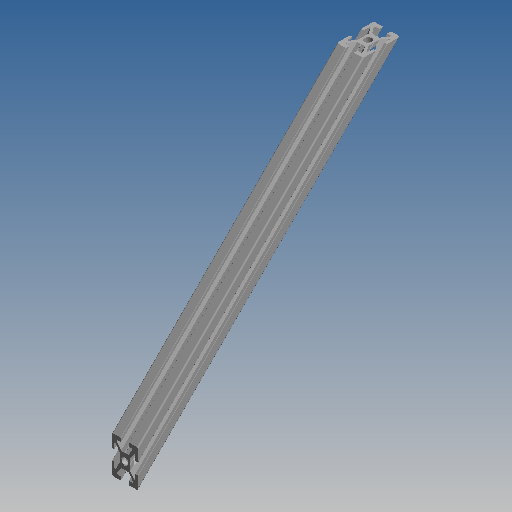
# Autodesk Inventor part: HFBL5-2020-200_
Saved by Autodesk Inventor 2020 (Build 240168000, 168)
## iProperties
Part Number: HFBL5-2020-200_
Material: 一般
Catalog Web Link: www.cadenas.de
Description: HFBL5_-Brackets HFS5 Frame Brackets for Reinforcement
Vendor: MISUMI
Document SubType Name: Modeling
Designer: partserver
Manufacturer: MISUMI
Mass: 47.3793 g
Surface Area: 458.252 cm^2
Volume: 47.3793 cm^3
Density: 1 g/cm^3
Appearance: PSOLRGB-192-192-192
Category: PARTsolutions
Company: MISUMI
PSOL_IDENT_0: {$CADENAS_DATA\23d-libs\misumi\metric\38_al_extrusions_blackets\5\hfbl5.prj},176 {VTYP=3D},{NB=HFBL5
PSOL_IDENT_1: -2020-200_},{LINA=HFBL5-2020-200_},{NN=HFBL5_},{DATE=24.04.2017 10:22:18},{GEOMDATE=30.01.2015 00:00
PSOL_IDENT_2: :00},{VERSION=},{LINEID=10},{WBVAR=L,ALT},{WBNUMERIC=L}  {NB=HFBL5-2020-200_},{LINA=HFBL5-2020-200_}
PSOL_IDENT_3: ,{KT=1},{PN=HFBL5-2020-200},{TP=HFBL5},{NO=2020},{TYPE=HFBL5},{MAT=A6N01SS-T5},{ST=Alumite Treatment
PSOL_IDENT_4: (No surface treatment on the side cut at 45 degree and  Counterbore type)},{FEAT=4 Slots},{L=200},{
PSOL_IDENT_5: LTOL=+/- 0.5},{MASS=0.50},{SA=153},{GMILX=0.57x10^4},{GMILY=0.57x10^4},{WIDTH=20},{HEIGHT=20},{TAPDE
PSOL_IDENT_6: PTH=15},{TAPSTART=0},{DRILLLENGTH=0},{DRILLDIA=4.2},{TAPPOSHOR=0},{TAPPOSVER=0},{VER=1},{DIM=1},{CLF=
PSOL_IDENT_7: HFS5-2020},{ALT3=},{AB=CBM5-8},{ABQ=2},{AN=HNTT5-5},{ANQ=2},{ALT=}
NB: HFBL5-2020-200_
NN: HFBL5_
NT: Brackets HFS5 Frame Brackets for Reinforcement
NBSYN: $PN._
LINA: HFBL5-2020-200_
CATALOG: Misumi
PN: HFBL5-2020-200
NO: 2020
MAT: A6N01SS-T5 Aluminum Alloy
ST: Alumite Treatment (No surface treatment on the side cut at 45 degree and  Counterbore type)
L: 200
WIDTH: 20
AB: CBM5-8
ABQ: 2
AN: HNTT5-5
ANQ: 2
ALT: w/o Set of Applicable Bolt and Nut
SUPPLIER: MISUMI
ARTICLENO: HFBL5-2020-200_
BOMINFO: HFBL5-2020-200_
CREATOR: CADENAS GmbH
Title: HFBL5-2020-200_
Author: Cadenas PARTsolutions
Comments: Brackets HFS5 Frame Brackets for Reinforcement
Autodesk Inventor part; units mm, degrees
sketch "Sketch_1" plane through (0, 0, 0) normal (0, -0.7071068, 0.7071068) x (1, 0, 0)
  arc A0 (-10, 134.7214) -> (-9.7, 134.4214) centre (-9.7, 134.7214) ccw
  line L0 (-9.7, 134.4214) -> (-8, 134.4214)
  line L1 (-8, 134.4214) -> (-8, 137.4214)
  line L2 (-8, 137.4214) -> (-7.0607, 137.4214)
  line L3 (-7.0607, 137.4214) -> (-4, 134.3607)
  line L4 (-4, 134.3607) -> (-4, 131.7214)
  line L5 (-4, 131.7214) -> (-3.7, 131.4214)
  line L6 (-3.7, 131.4214) -> (-4, 131.1214)
  line L7 (-4, 131.1214) -> (-4, 128.482)
  line L8 (-4, 128.482) -> (-7.0607, 125.4214)
  line L9 (-7.0607, 125.4214) -> (-8, 125.4214)
  line L10 (-8, 125.4214) -> (-8, 128.4214)
  line L11 (-8, 128.4214) -> (-9.7, 128.4214)
  arc A1 (-9.7, 128.4214) -> (-10, 128.1214) centre (-9.7, 128.1214) ccw
  line L12 (-10, 128.1214) -> (-10, 122.4214)
  arc A2 (-10, 122.4214) -> (-9, 121.4214) centre (-9, 122.4214) ccw
  line L13 (-9, 121.4214) -> (-3.3, 121.4214)
  arc A3 (-3.3, 121.4214) -> (-3, 121.7214) centre (-3.3, 121.7214) ccw
  line L14 (-3, 121.7214) -> (-3, 123.4214)
  line L15 (-3, 123.4214) -> (-6, 123.4214)
  line L16 (-6, 123.4214) -> (-6, 124.3607)
  line L17 (-6, 124.3607) -> (-2.9393, 127.4214)
  line L18 (-2.9393, 127.4214) -> (-0.3, 127.4214)
  line L19 (-0.3, 127.4214) -> (0, 127.7214)
  line L20 (0, 127.7214) -> (0.3, 127.4214)
  line L21 (0.3, 127.4214) -> (2.9393, 127.4214)
  line L22 (2.9393, 127.4214) -> (6, 124.3607)
  line L23 (6, 124.3607) -> (6, 123.4214)
  line L24 (6, 123.4214) -> (3, 123.4214)
  line L25 (3, 123.4214) -> (3, 121.7214)
  arc A4 (3, 121.7214) -> (3.3, 121.4214) centre (3.3, 121.7214) ccw
  line L26 (3.3, 121.4214) -> (9, 121.4214)
  arc A5 (9, 121.4214) -> (10, 122.4214) centre (9, 122.4214) ccw
  line L27 (10, 122.4214) -> (10, 128.1214)
  arc A6 (10, 128.1214) -> (9.7, 128.4214) centre (9.7, 128.1214) ccw
  line L28 (9.7, 128.4214) -> (8, 128.4214)
  line L29 (8, 128.4214) -> (8, 125.4214)
  line L30 (8, 125.4214) -> (7.0607, 125.4214)
  line L31 (7.0607, 125.4214) -> (4, 128.482)
  line L32 (4, 128.482) -> (4, 131.1214)
  line L33 (4, 131.1214) -> (3.7, 131.4214)
  line L34 (3.7, 131.4214) -> (4, 131.7214)
  line L35 (4, 131.7214) -> (4, 134.3607)
  line L36 (4, 134.3607) -> (7.0607, 137.4214)
  line L37 (7.0607, 137.4214) -> (8, 137.4214)
  line L38 (8, 137.4214) -> (8, 134.4214)
  line L39 (8, 134.4214) -> (9.7, 134.4214)
  arc A7 (9.7, 134.4214) -> (10, 134.7214) centre (9.7, 134.7214) ccw
  line L40 (10, 134.7214) -> (10, 140.4214)
  arc A8 (10, 140.4214) -> (9, 141.4214) centre (9, 140.4214) ccw
  line L41 (9, 141.4214) -> (3.3, 141.4214)
  arc A9 (3.3, 141.4214) -> (3, 141.1214) centre (3.3, 141.1214) ccw
  line L42 (3, 141.1214) -> (3, 139.4214)
  line L43 (3, 139.4214) -> (6, 139.4214)
  line L44 (6, 139.4214) -> (6, 138.482)
  line L45 (6, 138.482) -> (2.9393, 135.4214)
  line L46 (2.9393, 135.4214) -> (0.3, 135.4214)
  line L47 (0.3, 135.4214) -> (0, 135.1214)
  line L48 (0, 135.1214) -> (-0.3, 135.4214)
  line L49 (-0.3, 135.4214) -> (-2.9393, 135.4214)
  line L50 (-2.9393, 135.4214) -> (-6, 138.482)
  line L51 (-6, 138.482) -> (-6, 139.4214)
  line L52 (-6, 139.4214) -> (-3, 139.4214)
  line L53 (-3, 139.4214) -> (-3, 141.1214)
  arc A10 (-3, 141.1214) -> (-3.3, 141.4214) centre (-3.3, 141.1214) ccw
  line L54 (-3.3, 141.4214) -> (-9, 141.4214)
  arc A11 (-9, 141.4214) -> (-10, 140.4214) centre (-9, 140.4214) ccw
  line L55 (-10, 140.4214) -> (-10, 134.7214)
  circle A12 centre (0, 131.4214) radius 2.1
  constraints: 112 end point, 24 point on circle, 13 centre point
extrude "Extrusion1" add sketch "Sketch_1" along normal mid plane 284.8427
sketch "Sketch_2" plane through (0, 0, 0) normal (0, 0, 1) x (1, 0, 0)
  line L0 (-50, -300) -> (50, -300)
  line L1 (50, -300) -> (50, 0)
  line L2 (50, 0) -> (-50, 0)
  line L3 (-50, 0) -> (-50, -300)
  constraints: 8 end point
extrude "Extrusion2" cut sketch "Sketch_2" along normal mid plane 800
sketch "Sketch_3" plane through (0, 0, 0) normal (0, 1, 0) x (-1, 0, 0)
  line L0 (50, -300) -> (50, 0)
  line L1 (50, 0) -> (-50, 0)
  line L2 (-50, 0) -> (-50, -300)
  line L3 (-50, -300) -> (50, -300)
  constraints: 8 end point
extrude "Extrusion3" cut sketch "Sketch_3" along normal mid plane 800
sketch "Sketch_4" plane through (0, 0, 0) normal (1, 0, 0) x (0, 1, 0)
  line L0 (0, 185.65) -> (30, 185.65)
  line L1 (30, 185.65) -> (30, 180.9)
  line L2 (30, 180.9) -> (3, 180.9)
  line L3 (3, 180.9) -> (3, 182.9)
  line L4 (3, 182.9) -> (0, 182.9)
  line L5 (0, 182.9) -> (0, 185.65)
  line L6 (0, 185.65) -> (30, 185.65)
  constraints: 14 end point
revolve "Revolution1" cut sketch "Sketch_4" angle 360 about axis through (0, 0, 185.65) along (0, -1, 0)
sketch "Sketch_5" plane through (0, 0, 0) normal (1, 0, 0) x (0, 1, 0)
  line L0 (185.65, 0) -> (185.65, 30)
  line L1 (185.65, 30) -> (190.4, 30)
  line L2 (190.4, 30) -> (190.4, 3)
  line L3 (190.4, 3) -> (188.4, 3)
  line L4 (188.4, 3) -> (188.4, 0)
  line L5 (188.4, 0) -> (185.65, 0)
  line L6 (185.65, 0) -> (185.65, 30)
  constraints: 14 end point
revolve "Revolution2" cut sketch "Sketch_5" angle 360 about axis through (0, 185.65, 0) along (0, 0, -1)
ref_plane "bolt1_XY" through (0, 3, 185.65) normal (0, 1, 0) x (1, 0, 0)
ref_plane "bolt1_YZ" through (0, 3, 185.65) normal (1, 0, 0) x (0, 0, -1)
ref_plane "bolt1_ZX" through (0, 3, 185.65) normal (0, 0, -1) x (0, 1, 0)
ref_plane "bolt2_XY" through (0, 185.65, 3) normal (0, 0, 1) x (1, 0, 0)
ref_plane "bolt2_YZ" through (0, 185.65, 3) normal (1, 0, 0) x (0, 1, 0)
ref_plane "bolt2_ZX" through (0, 185.65, 3) normal (0, 1, 0) x (0, 0, 1)
body "Solid1"
